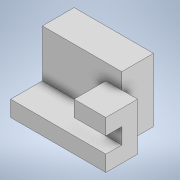
# Autodesk Inventor part: 零件11
Saved by Autodesk Inventor 2020 (Build 240168000, 168)
## iProperties
Created: 2020-09-19
Part Number: 零件11
Material: 一般
Document SubType Name: Modeling
Designer: User
Density: 1 g/cm^3
Appearance: 預設
Author: User
Autodesk Inventor part; units mm, degrees
ref_plane "YZ Plane" through (0, 0, 0) normal (1, 0, 0) x (0, 1, 0)
ref_plane "XZ Plane" through (0, 0, 0) normal (0, 1, 0) x (-1, 0, 0)
ref_plane "XY Plane" through (0, 0, 0) normal (0, 0, 1) x (1, 0, 0)
sketch "草圖1" plane through (0, 0, 0) normal (1, 0, 0) x (0, 1, 0)
  line L0 (0, 0) -> (40, 0)
  line L1 (40, 0) -> (40, -20)
  line L2 (40, -20) -> (0, -20)
  line L3 (0, -20) -> (0, 0)
  line L4 (0, 0) -> (30, 0)
  line L5 (30, 0) -> (30, 20)
  line L6 (0, 20) -> (0, 0)
  line L7 (10, 20) -> (20, 20)
  line L8 (20, 20) -> (20, 10)
  line L9 (20, 10) -> (10, 10)
  line L10 (10, 10) -> (10, 20)
  line L11 (10, 10) -> (10, 0)
  line L12 (30, 20) -> (20, 20)
  line L13 (10, 20) -> (0, 20)
  dimension "d0" = 40
  dimension "d1" = 20
  dimension "d2" = 30
  dimension "d3" = 20
  dimension "d4" = 10
  dimension "d5" = 10
  dimension "d6" = 10
  constraints: 28 end point, 7 parallel, 4 perpendicular, 3 horizontal, 1 point on line
  measures "d0" distance of L1.end L2.end
  measures "d1" distance of L0.end L1.end
  measures "d2" distance of L6.start L5.end
  measures "d3" distance of L5.end L4.end
  measures "d4" distance of L8.end L9.end
  measures "d5" distance of L7.end L8.end
  measures "d6" distance between parallel lines of L8 L5
extrude "擠出1" add sketch "草圖1" against normal blind 50 contours L6 L13 L10 L11 L0 | L0 L1 L2 L3
extrude "擠出2" add sketch "草圖1" against normal mid plane 20 contours L6 L13 L10 L11 L0 | L11 L9 L8 L12 L5 L0
